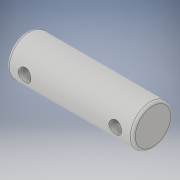
# Autodesk Inventor part: Crankshaft Center Rod
Saved by Autodesk Inventor 2017 (Build 210142000, 142)
## iProperties
Created: 2018-10-30
Part Number: Crankshaft Center Rod
Material: Generic
Document SubType Name: Modeling
Designer: 623516
Density: 1 g/cm^3
Appearance: Default
Author: 623516
Autodesk Inventor part; units mm, degrees
ref_plane "YZ Plane" through (0, 0, 0) normal (1, 0, 0) x (0, 1, 0)
ref_plane "XZ Plane" through (0, 0, 0) normal (0, 1, 0) x (-1, 0, 0)
sketch "Sketch1" plane through (0, 0, 0) normal (1, 0, 0) x (0, 1, 0)
  circle A0 centre (0, 0) radius 4
  dimension "d0" = 8
  constraints: 1 centre point, 1 coincident
  measures "d0" diameter of A0
extrude "Extrusion1" add sketch "Sketch1" along normal blind 25
fillet "Fillet1" radius 0.5 2 edges at (0, -4, 0) (25, -4, 0)
ref_plane "Work Plane1" through (0, 0, 4.7625) normal (0, 0, 1) x (1, 0, 0)
sketch "Sketch2" plane through (0, 0, 4.7625) normal (0, 0, 1) x (1, 0, 0)
  line L0 (0.5, 4) -> (24.5, 4) construction
  line L1 (12.5, 4) -> (12.5, 0) construction
  line L2 (12.5, 0) -> (21.5, 0) construction
  circle A0 centre (21.5, 0) radius 1.25 construction
  line L3 (12.5, 0) -> (3.5, 0) construction
  circle A1 centre (3.5, 0) radius 1.25 construction
  circle A2 centre (3.5, 0) radius 1.25
  circle A3 centre (21.5, 0) radius 1.25
  point P0 (0, 0)
  dimension "d5" = 9
  dimension "d6" = 2.5
  dimension "d7" = 9
  dimension "d8" = 2.5
  dimension "d9" = 4
  constraints: 6 end point, 4 centre point, 4 coincident, 2 equal radius, 1 horizontal, 1 midpoint, 1 perpendicular, 1 vertical
  measures "d5" distance of L1.end L2.end
  measures "d6" diameter of A0
  measures "d7" distance of L1.end L3.end
  measures "d8" diameter of A1
  measures "d9" distance between parallel lines of L2 L0
extrude "Extrusion2" cut sketch "Sketch2" against normal blind 25
body "Solid1"
